Autodesk Fusion 360 part; units mm, degrees
(part 5 of 5)
sketch "Boceto9" plane through (0, 4.8, 0) normal (0, 1, 0) x (-1, 0, 0)
  line L0 (-13.4347, -89.9523) -> (-1.4347, -77.5976)
  arc A0 (1.4347, -77.5976) -> (-1.4347, -77.5976) centre (0, -78.991) ccw
  line L1 (1.4347, -77.5976) -> (13.4347, -89.9523)
  arc A1 (12, -93.3458) -> (13.4347, -89.9523) centre (12, -91.3458) ccw
  line L2 (12, -93.3458) -> (-12, -93.3458)
  arc A2 (-13.4347, -89.9523) -> (-12, -93.3458) centre (-12, -91.3458) ccw
  line L3 (13.0951, -76.1205) -> (19, -76.1205)
  arc A3 (21, -78.1205) -> (19, -76.1205) centre (19, -78.1205) ccw
  line L4 (21, -78.1205) -> (21, -84.2)
  arc A4 (17.5653, -85.5935) -> (21, -84.2) centre (19, -84.2) ccw
  line L5 (17.5653, -85.5935) -> (11.6604, -79.514)
  arc A5 (13.0951, -76.1205) -> (11.6604, -79.514) centre (13.0951, -78.1205) ccw
  line L6 (-11.6604, -79.514) -> (-17.5653, -85.5935)
  arc A6 (-21, -84.2) -> (-17.5653, -85.5935) centre (-19, -84.2) ccw
  line L7 (-21, -84.2) -> (-21, -78.1205)
  arc A7 (-19, -76.1205) -> (-21, -78.1205) centre (-19, -78.1205) ccw
  line L8 (-19, -76.1205) -> (-13.0951, -76.1205)
  arc A8 (-11.6604, -79.514) -> (-13.0951, -76.1205) centre (-13.0951, -78.1205) ccw
  line L9 (8, -66.3205) -> (8, -67.1205)
  arc A9 (5, -70.1205) -> (8, -67.1205) centre (5, -67.1205) ccw
  line L10 (5, -70.1205) -> (-5, -70.1205)
  arc A10 (-8, -67.1205) -> (-5, -70.1205) centre (-5, -67.1205) ccw
  line L11 (-8, -67.1205) -> (-8, -66.3205)
  arc A11 (-5, -63.3205) -> (-8, -66.3205) centre (-5, -66.3205) ccw
  line L12 (-5, -63.3205) -> (5, -63.3205)
  arc A12 (8, -66.3205) -> (5, -63.3205) centre (5, -66.3205) ccw
  circle A13 centre (138.0313, 4.5) radius 2.5
  circle A14 centre (-140.0313, 14.5) radius 4
  arc A15 (124.6679, -20.512) -> (128.2, -19.2264) centre (126.2, -19.2264) ccw
  line L13 (124.6679, -20.512) -> (114.4087, -8.2856)
  arc A16 (115.9408, -5) -> (114.4087, -8.2856) centre (115.9408, -7) ccw
  line L14 (115.9408, -5) -> (126.2, -5)
  arc A17 (128.2, -7) -> (126.2, -5) centre (126.2, -7) ccw
  line L15 (128.2, -7) -> (128.2, -19.2264)
  arc A18 (-114.4087, -8.2856) -> (-115.9408, -5) centre (-115.9408, -7) ccw
  line L16 (-114.4087, -8.2856) -> (-124.6679, -20.512)
  arc A19 (-128.2, -19.2264) -> (-124.6679, -20.512) centre (-126.2, -19.2264) ccw
  line L17 (-128.2, -19.2264) -> (-128.2, -7)
  arc A20 (-126.2, -5) -> (-128.2, -7) centre (-126.2, -7) ccw
  line L18 (-126.2, -5) -> (-115.9408, -5)
  circle A21 centre (-143.9289, -24) radius 2.5
  arc A22 (131.7, 16.1564) -> (129.934, 16.7992) centre (130.7, 16.1564) ccw
  line L19 (131.7, 16.1564) -> (131.7, 1)
  arc A23 (130.7, 0) -> (131.7, 1) centre (130.7, 1) ccw
  line L20 (130.7, 0) -> (117.9823, 0)
  arc A24 (117.2162, 1.6428) -> (117.9823, 0) centre (117.9823, 1) ccw
  line L21 (117.2162, 1.6428) -> (129.934, 16.7992)
  arc A25 (-129.934, 16.7992) -> (-131.7, 16.1564) centre (-130.7, 16.1564) ccw
  line L22 (-129.934, 16.7992) -> (-117.2162, 1.6428)
  arc A26 (-117.9823, 0) -> (-117.2162, 1.6428) centre (-117.9823, 1) ccw
  line L23 (-117.9823, 0) -> (-130.7, 0)
  arc A27 (-131.7, 1) -> (-130.7, 0) centre (-130.7, 1) ccw
  line L24 (-131.7, 1) -> (-131.7, 16.1564)
  circle A28 centre (143.9289, -24) radius 2.5
  circle A29 centre (-138.0313, 4.5) radius 2.5
  circle A30 centre (140.0313, 14.5) radius 4
  line L25 (23, -57.3205) -> (-23, -57.3205)
  line L26 (-23, -57.3205) -> (-23, -5)
  line L27 (-23, -5) -> (23, -5)
  line L28 (23, -5) -> (23, -57.3205)
  line L29 (30, -92.2) -> (122.2222, -25.3759)
  line L30 (122.2222, -25.3759) -> (126.7013, -30.7139)
  arc A31 (126.7013, -30.7139) -> (130.5315, -32.5) centre (130.5315, -27.5) ccw
  line L31 (130.5315, -32.5) -> (131.95, -32.5)
  line L32 (131.95, -32.5) -> (133.2, -31.25)
  line L33 (133.2, -31.25) -> (133.2, -5)
  line L34 (133.2, -5) -> (138, -5)
  line L35 (138, -5) -> (138, -31.5)
  line L36 (138, -31.5) -> (139, -32.5)
  line L37 (139, -32.5) -> (141.0289, -32.5)
  arc A32 (141.0289, -32.5) -> (149.6891, -17.5) centre (141.0289, -22.5) ccw
  arc A33 (148.5274, 15.3125) -> (149.6891, -17.5) centre (180, 0) ccw
  arc A34 (148.5274, 15.3125) -> (144.0313, 22.5) centre (144.0313, 17.5) ccw
  line L38 (144.0313, 22.5) -> (131.9209, 22.5)
  arc A35 (131.9209, 22.5) -> (125.7926, 19.6423) centre (131.9209, 14.5) ccw
  line L39 (125.7926, 19.6423) -> (115.9041, 7.8577)
  arc A36 (109.7758, 5) -> (115.9041, 7.8577) centre (109.7758, 13) ccw
  line L40 (109.7758, 5) -> (35, 5)
  arc A37 (30, 10) -> (35, 5) centre (35, 10) ccw
  line L41 (30, 10) -> (30, 12.6048)
  arc A38 (30, 12.6048) -> (26.8657, 15.6018) centre (27, 12.6048) ccw
  arc A39 (22.4813, 15.4213) -> (26.8657, 15.6018) centre (0, 615) ccw
  arc A40 (22.4813, 15.4213) -> (22, 14.9217) centre (22.5, 14.9217) ccw
  line L42 (22, 14.9217) -> (22, 8)
  line L43 (22, 8) -> (17.2, 8)
  line L44 (17.2, 8) -> (17.2, 14.7323)
  arc A41 (17.2, 14.7323) -> (16.6861, 15.2321) centre (16.7, 14.7323) ccw
  arc A42 (-8.6105, 15.0618) -> (16.6861, 15.2321) centre (0, 615) ccw
  line L45 (-8.6105, 15.0618) -> (-4.2286, 3.0227)
  arc A43 (-4.2286, 3.0227) -> (0, 9.0618) centre (0, 4.5618) ccw
  arc A44 (0, 11.0618) -> (0, 9.0618) centre (0, 10.0618) ccw
  arc A45 (-6.108, 2.3387) -> (0, 11.0618) centre (0, 4.5618) ccw
  line L46 (-6.108, 2.3387) -> (-10.7514, 15.0963)
  arc A46 (-16.6861, 15.2321) -> (-10.7514, 15.0963) centre (0, 615) ccw
  arc A47 (-16.6861, 15.2321) -> (-17.2, 14.7323) centre (-16.7, 14.7323) ccw
  line L47 (-17.2, 14.7323) -> (-17.2, 8)
  line L48 (-17.2, 8) -> (-22, 8)
  line L49 (-22, 8) -> (-22, 14.9217)
  arc A48 (-22, 14.9217) -> (-22.4813, 15.4213) centre (-22.5, 14.9217) ccw
  arc A49 (-26.8657, 15.6018) -> (-22.4813, 15.4213) centre (0, 615) ccw
  arc A50 (-26.8657, 15.6018) -> (-30, 12.6048) centre (-27, 12.6048) ccw
  line L50 (-30, 12.6048) -> (-30, 10)
  arc A51 (-35, 5) -> (-30, 10) centre (-35, 10) ccw
  line L51 (-35, 5) -> (-109.7758, 5)
  arc A52 (-115.9041, 7.8577) -> (-109.7758, 5) centre (-109.7758, 13) ccw
  line L52 (-115.9041, 7.8577) -> (-125.7926, 19.6423)
  arc A53 (-125.7926, 19.6423) -> (-131.9209, 22.5) centre (-131.9209, 14.5) ccw
  line L53 (-131.9209, 22.5) -> (-144.0313, 22.5)
  arc A54 (-144.0313, 22.5) -> (-148.5274, 15.3125) centre (-144.0313, 17.5) ccw
  arc A55 (-149.6891, -17.5) -> (-148.5274, 15.3125) centre (-180, 0) ccw
  arc A56 (-149.6891, -17.5) -> (-141.0289, -32.5) centre (-141.0289, -22.5) ccw
  line L54 (-141.0289, -32.5) -> (-139, -32.5)
  line L55 (-139, -32.5) -> (-138, -31.5)
  line L56 (-138, -31.5) -> (-138, -5)
  line L57 (-138, -5) -> (-133.2, -5)
  line L58 (-133.2, -5) -> (-133.2, -31.25)
  line L59 (-133.2, -31.25) -> (-131.95, -32.5)
  line L60 (-131.95, -32.5) -> (-130.5315, -32.5)
  arc A57 (-130.5315, -32.5) -> (-126.7013, -30.7139) centre (-130.5315, -27.5) ccw
  line L61 (-126.7013, -30.7139) -> (-122.2222, -25.3759)
  line L62 (-122.2222, -25.3759) -> (-30, -92.2)
  line L63 (-30, -92.2) -> (-20, -92.2)
  line L64 (-20, -92.2) -> (-20, -97)
  line L65 (-20, -97) -> (-30, -97)
  line L66 (-30, -97) -> (-30, -101)
  arc A58 (-30, -101) -> (-26, -105) centre (-26, -101) ccw
  line L67 (-26, -105) -> (-10, -105)
  line L68 (-10, -105) -> (-0.8439, -100.7385)
  arc A59 (0.8439, -100.7385) -> (-0.8439, -100.7385) centre (0, -102.5518) ccw
  line L69 (0.8439, -100.7385) -> (10, -105)
  line L70 (10, -105) -> (26, -105)
  arc A60 (26, -105) -> (30, -101) centre (26, -101) ccw
  line L71 (30, -101) -> (30, -97)
  line L72 (30, -97) -> (20, -97)
  line L73 (20, -97) -> (20, -92.2)
  line L74 (20, -92.2) -> (30, -92.2)
  line L75 (30, -63.3205) -> (30, -7.5)
  arc A61 (32.5, -5) -> (30, -7.5) centre (32.5, -7.5) ccw
  line L76 (32.5, -5) -> (101.3943, -5)
  arc A62 (107.5227, -7.8577) -> (101.3943, -5) centre (101.3943, -13) ccw
  line L77 (107.5227, -7.8577) -> (117.7113, -20)
  line L78 (117.7113, -20) -> (30, -83.5555)
  line L79 (30, -83.5555) -> (30, -68.1205)
  line L80 (30, -68.1205) -> (16, -68.1205)
  line L81 (16, -68.1205) -> (16, -63.3205)
  line L82 (16, -63.3205) -> (30, -63.3205)
  line L83 (-30, -7.5) -> (-30, -63.3205)
  line L84 (-30, -63.3205) -> (-16, -63.3205)
  line L85 (-16, -63.3205) -> (-16, -68.1205)
  line L86 (-16, -68.1205) -> (-30, -68.1205)
  line L87 (-30, -68.1205) -> (-30, -83.5555)
  line L88 (-30, -83.5555) -> (-117.7113, -20)
  line L89 (-117.7113, -20) -> (-107.5227, -7.8577)
  arc A63 (-101.3943, -5) -> (-107.5227, -7.8577) centre (-101.3943, -13) ccw
  line L90 (-101.3943, -5) -> (-32.5, -5)
  arc A64 (-30, -7.5) -> (-32.5, -5) centre (-32.5, -7.5) ccw
  line L91 (-30, -63.3205) -> (-88.3205, -5)
  line L92 (-30, -52.0068) -> (-77.0068, -5)
  line L93 (0, 1.75) -> (0, 22.5)
  line L94 (30, -52.0068) -> (77.0068, -5)
  line L95 (30, -63.3205) -> (88.3205, -5)
  dimension "d158" = 8
  dimension "d159" = 45
  constraint coincident L83.end L84.start
  constraint coincident L90 L91.end
  constraint coincident L83 L92.start
  constraint coincident L90 L92.end
  constraint parallel L91 L92
  constraint symmetric L83.end L93 L75.start
  constraint symmetric L91.end L93 L95.end
  constraint symmetric L92.start L93 L94.start
  constraint symmetric L92.end L93 L94.end
  measures "d158" distance of L91 L92
  measures "d159" angle of L83 L92
extrude "Extruir8" add sketch "Boceto9" against normal blind 4.8 contours L75 L76 L94 L95 | L83 L90 L91 L92
chamfer "Chaflán3" distance 5 angle 45 4 edges at (23, 2.4, -57.3205) (23, 2.4, -5) (-23, 2.4, -57.3205) (-23, 2.4, -5)
fillet "Empalme7" radius 5 12 edges at (30, 2.4, -83.5555) (30, 2.4, -52.0068) (77.0068, 2.4, -5) (122.2222, 2.4, -25.3759) (117.7113, 2.4, -20) (-30, 2.4, -83.5555) (-30, 2.4, -52.0068) (-77.0068, 2.4, -5) (-117.7113, 2.4, -20) (-122.2222, 2.4, -25.3759) (-88.3205, 2.4, -5) (88.3205, 2.4, -5)
chamfer "Chaflán4" distance 1 angle 45 7 edges at (30, 2.4, -68.1205) (30, 2.4, -97) (-30, 2.4, -97) (-30, 2.4, -68.1205) (8.6105, 2.4, 15.0618) (30, 2.4, -63.3205) (-30, 2.4, -63.3205)
sketch "Boceto11" plane through (0, 4.8, 0) normal (0, 1, 0) x (-1, 0, 0)
  line L0 (29, -63.3205) -> (30.7071, -62.6134)
  line L1 (30.7071, -62.6134) -> (86.856, -6.4645)
  arc A0 (90.3916, -5) -> (86.856, -6.4645) centre (90.3916, -10) ccw
  line L2 (90.3916, -5) -> (101.3943, -5)
  arc A1 (107.5227, -7.8577) -> (101.3943, -5) centre (101.3943, -13) ccw
  line L3 (107.5227, -7.8577) -> (114.2603, -15.8873)
  arc A2 (113.3639, -23.1501) -> (114.2603, -15.8873) centre (110.4301, -19.1013) ccw
  line L4 (113.3639, -23.1501) -> (37.9338, -77.8067)
  arc A3 (30, -73.7579) -> (37.9338, -77.8067) centre (35, -73.7579) ccw
  line L5 (30, -73.7579) -> (30, -69.1205)
  line L6 (30, -69.1205) -> (29, -68.1205)
  line L7 (29, -68.1205) -> (16, -68.1205)
  line L8 (16, -68.1205) -> (16, -63.3205)
  line L9 (16, -63.3205) -> (29, -63.3205)
  line L10 (-30.7071, -62.6134) -> (-29, -63.3205)
  line L11 (-29, -63.3205) -> (-16, -63.3205)
  line L12 (-16, -63.3205) -> (-16, -68.1205)
  line L13 (-16, -68.1205) -> (-29, -68.1205)
  line L14 (-29, -68.1205) -> (-30, -69.1205)
  line L15 (-30, -69.1205) -> (-30, -73.7579)
  arc A4 (-37.9338, -77.8067) -> (-30, -73.7579) centre (-35, -73.7579) ccw
  line L16 (-37.9338, -77.8067) -> (-113.3639, -23.1501)
  arc A5 (-114.2603, -15.8873) -> (-113.3639, -23.1501) centre (-110.4301, -19.1013) ccw
  line L17 (-114.2603, -15.8873) -> (-107.5227, -7.8577)
  arc A6 (-101.3943, -5) -> (-107.5227, -7.8577) centre (-101.3943, -13) ccw
  line L18 (-101.3943, -5) -> (-90.3916, -5)
  arc A7 (-86.856, -6.4645) -> (-90.3916, -5) centre (-90.3916, -10) ccw
  line L19 (-86.856, -6.4645) -> (-30.7071, -62.6134)
  line L20 (30, -39.9357) -> (30, -7.5)
  arc A8 (32.5, -5) -> (30, -7.5) centre (32.5, -7.5) ccw
  line L21 (32.5, -5) -> (64.9357, -5)
  arc A9 (68.4713, -13.5355) -> (64.9357, -5) centre (64.9357, -10) ccw
  line L22 (68.4713, -13.5355) -> (38.5355, -43.4713)
  arc A10 (30, -39.9357) -> (38.5355, -43.4713) centre (35, -39.9357) ccw
  line L23 (18, -57.3205) -> (-18, -57.3205)
  line L24 (-18, -57.3205) -> (-23, -52.3205)
  line L25 (-23, -52.3205) -> (-23, -10)
  line L26 (-23, -10) -> (-18, -5)
  line L27 (-18, -5) -> (18, -5)
  line L28 (18, -5) -> (23, -10)
  line L29 (23, -10) -> (23, -52.3205)
  line L30 (23, -52.3205) -> (18, -57.3205)
  circle A11 centre (140.0313, 14.5) radius 4
  arc A12 (124.6679, -20.512) -> (128.2, -19.2264) centre (126.2, -19.2264) ccw
  line L31 (124.6679, -20.512) -> (114.4087, -8.2856)
  arc A13 (115.9408, -5) -> (114.4087, -8.2856) centre (115.9408, -7) ccw
  line L32 (115.9408, -5) -> (126.2, -5)
  arc A14 (128.2, -7) -> (126.2, -5) centre (126.2, -7) ccw
  line L33 (128.2, -7) -> (128.2, -19.2264)
  arc A15 (131.7, 16.1564) -> (129.934, 16.7992) centre (130.7, 16.1564) ccw
  line L34 (131.7, 16.1564) -> (131.7, 1)
  arc A16 (130.7, 0) -> (131.7, 1) centre (130.7, 1) ccw
  line L35 (130.7, 0) -> (117.9823, 0)
  arc A17 (117.2162, 1.6428) -> (117.9823, 0) centre (117.9823, 1) ccw
  line L36 (117.2162, 1.6428) -> (129.934, 16.7992)
  circle A18 centre (-143.9289, -24) radius 2.5
  circle A19 centre (-140.0313, 14.5) radius 4
  circle A20 centre (143.9289, -24) radius 2.5
  circle A21 centre (-138.0313, 4.5) radius 2.5
  arc A22 (-129.934, 16.7992) -> (-131.7, 16.1564) centre (-130.7, 16.1564) ccw
  line L37 (-129.934, 16.7992) -> (-117.2162, 1.6428)
  arc A23 (-117.9823, 0) -> (-117.2162, 1.6428) centre (-117.9823, 1) ccw
  line L38 (-117.9823, 0) -> (-130.7, 0)
  arc A24 (-131.7, 1) -> (-130.7, 0) centre (-130.7, 1) ccw
  line L39 (-131.7, 1) -> (-131.7, 16.1564)
  circle A25 centre (138.0313, 4.5) radius 2.5
  arc A26 (-114.4087, -8.2856) -> (-115.9408, -5) centre (-115.9408, -7) ccw
  line L40 (-114.4087, -8.2856) -> (-124.6679, -20.512)
  arc A27 (-128.2, -19.2264) -> (-124.6679, -20.512) centre (-126.2, -19.2264) ccw
  line L41 (-128.2, -19.2264) -> (-128.2, -7)
  arc A28 (-126.2, -5) -> (-128.2, -7) centre (-126.2, -7) ccw
  line L42 (-126.2, -5) -> (-115.9408, -5)
  line L43 (8, -66.3205) -> (8, -67.1205)
  arc A29 (5, -70.1205) -> (8, -67.1205) centre (5, -67.1205) ccw
  line L44 (5, -70.1205) -> (-5, -70.1205)
  arc A30 (-8, -67.1205) -> (-5, -70.1205) centre (-5, -67.1205) ccw
  line L45 (-8, -67.1205) -> (-8, -66.3205)
  arc A31 (-5, -63.3205) -> (-8, -66.3205) centre (-5, -66.3205) ccw
  line L46 (-5, -63.3205) -> (5, -63.3205)
  arc A32 (8, -66.3205) -> (5, -63.3205) centre (5, -66.3205) ccw
  line L47 (-11.6604, -79.514) -> (-17.5653, -85.5935)
  arc A33 (-21, -84.2) -> (-17.5653, -85.5935) centre (-19, -84.2) ccw
  line L48 (-21, -84.2) -> (-21, -78.1205)
  arc A34 (-19, -76.1205) -> (-21, -78.1205) centre (-19, -78.1205) ccw
  line L49 (-19, -76.1205) -> (-13.0951, -76.1205)
  arc A35 (-11.6604, -79.514) -> (-13.0951, -76.1205) centre (-13.0951, -78.1205) ccw
  line L50 (13.0951, -76.1205) -> (19, -76.1205)
  arc A36 (21, -78.1205) -> (19, -76.1205) centre (19, -78.1205) ccw
  line L51 (21, -78.1205) -> (21, -84.2)
  arc A37 (17.5653, -85.5935) -> (21, -84.2) centre (19, -84.2) ccw
  line L52 (17.5653, -85.5935) -> (11.6604, -79.514)
  arc A38 (13.0951, -76.1205) -> (11.6604, -79.514) centre (13.0951, -78.1205) ccw
  line L53 (-13.4347, -89.9523) -> (-1.4347, -77.5976)
  arc A39 (1.4347, -77.5976) -> (-1.4347, -77.5976) centre (0, -78.991) ccw
  line L54 (1.4347, -77.5976) -> (13.4347, -89.9523)
  arc A40 (12, -93.3458) -> (13.4347, -89.9523) centre (12, -91.3458) ccw
  line L55 (12, -93.3458) -> (-12, -93.3458)
  arc A41 (-13.4347, -89.9523) -> (-12, -93.3458) centre (-12, -91.3458) ccw
  line L56 (-64.9357, -5) -> (-32.5, -5)
  arc A42 (-30, -7.5) -> (-32.5, -5) centre (-32.5, -7.5) ccw
  line L57 (-30, -7.5) -> (-30, -39.9357)
  arc A43 (-38.5355, -43.4713) -> (-30, -39.9357) centre (-35, -39.9357) ccw
  line L58 (-38.5355, -43.4713) -> (-68.4713, -13.5355)
  arc A44 (-64.9357, -5) -> (-68.4713, -13.5355) centre (-64.9357, -10) ccw
  line L59 (-7.6106, 15.0483) -> (-8.2685, 14.1221)
  line L60 (-8.2685, 14.1221) -> (-4.2286, 3.0227)
  arc A45 (-4.2286, 3.0227) -> (0, 9.0618) centre (0, 4.5618) ccw
  arc A46 (0, 11.0618) -> (0, 9.0618) centre (0, 10.0618) ccw
  arc A47 (-6.108, 2.3387) -> (0, 11.0618) centre (0, 4.5618) ccw
  line L61 (-6.108, 2.3387) -> (-10.7514, 15.0963)
  arc A48 (-16.6861, 15.2321) -> (-10.7514, 15.0963) centre (0, 615) ccw
  arc A49 (-16.6861, 15.2321) -> (-17.2, 14.7323) centre (-16.7, 14.7323) ccw
  line L62 (-17.2, 14.7323) -> (-17.2, 8)
  line L63 (-17.2, 8) -> (-22, 8)
  line L64 (-22, 8) -> (-22, 14.9217)
  arc A50 (-22, 14.9217) -> (-22.4813, 15.4213) centre (-22.5, 14.9217) ccw
  arc A51 (-26.8657, 15.6018) -> (-22.4813, 15.4213) centre (0, 615) ccw
  arc A52 (-26.8657, 15.6018) -> (-30, 12.6048) centre (-27, 12.6048) ccw
  line L65 (-30, 12.6048) -> (-30, 10)
  arc A53 (-35, 5) -> (-30, 10) centre (-35, 10) ccw
  line L66 (-35, 5) -> (-109.7758, 5)
  arc A54 (-115.9041, 7.8577) -> (-109.7758, 5) centre (-109.7758, 13) ccw
  line L67 (-115.9041, 7.8577) -> (-125.7926, 19.6423)
  arc A55 (-125.7926, 19.6423) -> (-131.9209, 22.5) centre (-131.9209, 14.5) ccw
  line L68 (-131.9209, 22.5) -> (-144.0313, 22.5)
  arc A56 (-144.0313, 22.5) -> (-148.5274, 15.3125) centre (-144.0313, 17.5) ccw
  arc A57 (-149.6891, -17.5) -> (-148.5274, 15.3125) centre (-180, 0) ccw
  arc A58 (-149.6891, -17.5) -> (-141.0289, -32.5) centre (-141.0289, -22.5) ccw
  line L69 (-141.0289, -32.5) -> (-139, -32.5)
  line L70 (-139, -32.5) -> (-138, -31.5)
  line L71 (-138, -31.5) -> (-138, -5)
  line L72 (-138, -5) -> (-133.2, -5)
  line L73 (-133.2, -5) -> (-133.2, -31.25)
  line L74 (-133.2, -31.25) -> (-131.95, -32.5)
  line L75 (-131.95, -32.5) -> (-130.5315, -32.5)
  arc A59 (-130.5315, -32.5) -> (-126.7013, -30.7139) centre (-130.5315, -27.5) ccw
  line L76 (-126.7013, -30.7139) -> (-125.2154, -28.9431)
  arc A60 (-118.4514, -28.1082) -> (-125.2154, -28.9431) centre (-121.3852, -32.157) ccw
  line L77 (-118.4514, -28.1082) -> (-30, -92.2)
  line L78 (-30, -92.2) -> (-20, -92.2)
  line L79 (-20, -92.2) -> (-20, -97)
  line L80 (-20, -97) -> (-29, -97)
  line L81 (-29, -97) -> (-30, -98)
  line L82 (-30, -98) -> (-30, -101)
  arc A61 (-30, -101) -> (-26, -105) centre (-26, -101) ccw
  line L83 (-26, -105) -> (-10, -105)
  line L84 (-10, -105) -> (-0.8439, -100.7385)
  arc A62 (0.8439, -100.7385) -> (-0.8439, -100.7385) centre (0, -102.5518) ccw
  line L85 (0.8439, -100.7385) -> (10, -105)
  line L86 (10, -105) -> (26, -105)
  arc A63 (26, -105) -> (30, -101) centre (26, -101) ccw
  line L87 (30, -101) -> (30, -98)
  line L88 (30, -98) -> (29, -97)
  line L89 (29, -97) -> (20, -97)
  line L90 (20, -97) -> (20, -92.2)
  line L91 (20, -92.2) -> (30, -92.2)
  line L92 (30, -92.2) -> (118.4514, -28.1082)
  arc A64 (125.2154, -28.9431) -> (118.4514, -28.1082) centre (121.3852, -32.157) ccw
  line L93 (125.2154, -28.9431) -> (126.7013, -30.7139)
  arc A65 (126.7013, -30.7139) -> (130.5315, -32.5) centre (130.5315, -27.5) ccw
  line L94 (130.5315, -32.5) -> (131.95, -32.5)
  line L95 (131.95, -32.5) -> (133.2, -31.25)
  line L96 (133.2, -31.25) -> (133.2, -5)
  line L97 (133.2, -5) -> (138, -5)
  line L98 (138, -5) -> (138, -31.5)
  line L99 (138, -31.5) -> (139, -32.5)
  line L100 (139, -32.5) -> (141.0289, -32.5)
  arc A66 (141.0289, -32.5) -> (149.6891, -17.5) centre (141.0289, -22.5) ccw
  arc A67 (148.5274, 15.3125) -> (149.6891, -17.5) centre (180, 0) ccw
  arc A68 (148.5274, 15.3125) -> (144.0313, 22.5) centre (144.0313, 17.5) ccw
  line L101 (144.0313, 22.5) -> (131.9209, 22.5)
  arc A69 (131.9209, 22.5) -> (125.7926, 19.6423) centre (131.9209, 14.5) ccw
  line L102 (125.7926, 19.6423) -> (115.9041, 7.8577)
  arc A70 (109.7758, 5) -> (115.9041, 7.8577) centre (109.7758, 13) ccw
  line L103 (109.7758, 5) -> (35, 5)
  arc A71 (30, 10) -> (35, 5) centre (35, 10) ccw
  line L104 (30, 10) -> (30, 12.6048)
  arc A72 (30, 12.6048) -> (26.8657, 15.6018) centre (27, 12.6048) ccw
  arc A73 (22.4813, 15.4213) -> (26.8657, 15.6018) centre (0, 615) ccw
  arc A74 (22.4813, 15.4213) -> (22, 14.9217) centre (22.5, 14.9217) ccw
  line L105 (22, 14.9217) -> (22, 8)
  line L106 (22, 8) -> (17.2, 8)
  line L107 (17.2, 8) -> (17.2, 14.7323)
  arc A75 (17.2, 14.7323) -> (16.6861, 15.2321) centre (16.7, 14.7323) ccw
  arc A76 (-7.6106, 15.0483) -> (16.6861, 15.2321) centre (0, 615) ccw
equation "d8 = d7 / 2"
equation "d28 = d23"
equation "d32 = 27.5 mm + 5 mm"
equation "d45 = d44"
equation "d47 = d46"
equation "d51 = 60 mm"
equation "d52 = d51 / 2"
equation "d65 = d67"
equation "d102 = d103"
equation "d112 = d102"
equation "d152 = d153"

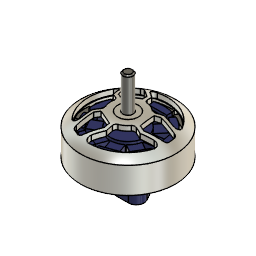
design "1102 BRUSHLESS"
Autodesk Fusion 360 part; units mm, degrees
sketch "Boceto1" plane through (0, 0, 0) normal (0, 0, 1) x (1, 0, 0)
  line L0 (-3.847, -1.0789) -> (-0.9891, 3.8711)
  line L1 (0.9891, 3.8711) -> (3.847, -1.0789)
  line L2 (2.8579, -2.7921) -> (-2.8579, -2.7921)
  line L3 (0, -2.7921) -> (0, 5.9712) construction
  line L4 (-2.5255, 1.2099) -> (5.4503, -2.6111) construction
  circle A0 centre (0, 3.3) radius 0.7
  circle A1 centre (0, 0) radius 3.3 construction
  arc A2 (0.9891, 3.8711) -> (-0.9891, 3.8711) centre (0, 3.3) ccw
  circle A3 centre (-2.8579, -1.65) radius 0.7
  arc A4 (-3.847, -1.0789) -> (-2.8579, -2.7921) centre (-2.8579, -1.65) ccw
  circle A5 centre (2.8579, -1.65) radius 0.7
  arc A6 (2.8579, -2.7921) -> (3.847, -1.0789) centre (2.8579, -1.65) ccw
  line L5 (-4, -1.65) -> (4, -1.65) construction
  line L6 (4, -1.65) -> (4, -0.8) construction
  dimension "d3" = 6.6
  dimension "d4" = 1.4
  dimension "d7" = 360
  dimension "d8" = 8
  constraint horizontal L2
  constraint vertical L3
  constraint coincident A1.centre L3
  constraint coincident A1.centre L4
  constraint coincident L3 A0.centre
  constraint coincident A1.centre origin
  constraint coincident A0.centre A1
  constraint tangent L1 A2
  constraint coincident L0 L4.start
  constraint concentric A0 A2
  constraint coincident A4 L2.end
  constraint coincident L2 L3.start
  constraint coincident A6 L2.start
  constraint coincident L1.end A6.end
  constraint tangent L0 A2
  constraint coincident A4 L5.start
  constraint coincident A6 L5.end
  constraint horizontal L5
  constraint coincident L2.start A6.start
  constraint perpendicular L5 L6
  constraint tangent A6 L6
  measures "d3" diameter of A1
  measures "d4" diameter of A0
  measures "d8" distance of L5.start L5.end
extrude "Extruir1" add sketch "Boceto1" along normal blind 1.25 makes body 1
sketch "Boceto2" plane through (0, 0, 1.25) normal (0, 0, 1) x (-1, 0, 0)
  circle A0 centre (2.8579, 1.65) radius 0.7
  circle A1 centre (0, -3.3) radius 0.7
  circle A2 centre (-2.8579, 1.65) radius 0.7
  arc A3 (3.847, 1.0789) -> (2.8579, 2.7921) centre (2.8579, 1.65) ccw
  line L0 (2.8579, 2.7921) -> (-2.8579, 2.7921)
  arc A4 (-2.8579, 2.7921) -> (-3.847, 1.0789) centre (-2.8579, 1.65) ccw
  line L1 (-3.847, 1.0789) -> (-0.9891, -3.8711)
  arc A5 (-0.9891, -3.8711) -> (0.9891, -3.8711) centre (0, -3.3) ccw
  line L2 (0.9891, -3.8711) -> (3.847, 1.0789)
  circle A6 centre (0, 0) radius 2.6
  constraint coincident A6.centre origin
  constraint tangent A1 A6
extrude "Extruir2" add sketch "Boceto2" along normal blind 5.5 contours A6 bodies 1
sketch "Boceto3" plane through (0, 0, 0) normal (0, 0, -1) x (1, 0, 0)
  circle A0 centre (-2.8579, 1.65) radius 0.7
  circle A1 centre (0, -3.3) radius 0.7
  circle A2 centre (2.8579, 1.65) radius 0.7
  arc A3 (-2.8579, 2.7921) -> (-3.847, 1.0789) centre (-2.8579, 1.65) ccw
  line L0 (-3.847, 1.0789) -> (-0.9891, -3.8711)
  arc A4 (-0.9891, -3.8711) -> (0.9891, -3.8711) centre (0, -3.3) ccw
  line L1 (0.9891, -3.8711) -> (3.847, 1.0789)
  arc A5 (3.847, 1.0789) -> (2.8579, 2.7921) centre (2.8579, 1.65) ccw
  line L2 (2.8579, 2.7921) -> (-2.8579, 2.7921)
  circle A6 centre (0, 0) radius 2
  dimension "d14" = 4
  constraint coincident A6.centre origin
  measures "d14" diameter of A6
extrude "Extruir3" cut sketch "Boceto3" against normal blind 1 contours A6 bodies 1
sketch "Boceto4" plane through (0, 0, 1) normal (0, 0, -1) x (1, 0, 0)
  circle A0 centre (0, 0) radius 2
  circle A1 centre (0, 0) radius 0.75
  dimension "d17" = 1.5
  constraint coincident A0.centre A1.centre
  measures "d17" diameter of A1
extrude "Extruir4" cut sketch "Boceto4" against normal blind 10 contours A1 bodies 1
extrude "Extruir5" add 1 faces at (1.5731, 0.1366, 1) along direction (0, 0, -1) blind 1 separate body on bodies 1 makes body 2
sketch "Boceto5" plane through (0, 0, 0) normal (0, 0, -1) x (1, 0, 0)
  circle A0 centre (0, 0) radius 0.75
  circle A1 centre (0, 0) radius 2
extrude "Extruir6" add sketch "Boceto5" against normal blind 13.75 separate body contours A0 makes body 3
extrude "Extruir8" add 1 faces at (0.5555, 0.0837, 0) along direction (0, 0, -1) blind 0.5 on bodies 3 bodies 3
ref_plane "PlanoDeObra1" through (0, 2.6, 5.2604) normal (0, 1, 0) x (1, 0, 0)
sketch "Boceto7" plane through (0, 2.6, 0) normal (0, 1, 0) x (1, 0, 0)
  line L0 (0.85, -6.35) -> (-0.85, -6.35)
  line L1 (-0.85, -6.35) -> (-0.85, -4.05)
  line L2 (-0.85, -4.05) -> (0.85, -4.05)
  line L3 (0.85, -4.05) -> (0.85, -6.35)
  line L4 (-2.6, -6.75) -> (2.6, -6.75)
  line L5 (0, -4.05) -> (0, -6.35) construction
  dimension "d30" = 1.7
  dimension "d31" = 2.3
  dimension "d42" = 0.4
  constraint horizontal L0
  constraint vertical L1
  constraint horizontal L2
  constraint vertical L3
  constraint midpoint L2 L5.start
  constraint midpoint L0 L5.end
  constraint coincident origin L5
  constraint coincident L0.end L1.start
  measures "d30" distance of L0.start L0.end
  measures "d31" distance of L0.start L2.end
  measures "d42" distance of L0 L4
extrude "Extruir9" add sketch "Boceto7" along normal blind 1.7 and the other way blind 0.5 bodies 1
sketch "Boceto8" plane through (0, 4.3, 0) normal (0, 1, 0) x (-1, 0, 0)
  line L0 (0.85, 6.35) -> (-0.85, 6.35)
  line L1 (-0.85, 6.35) -> (-0.85, 4.05)
  line L2 (-0.85, 4.05) -> (0.85, 4.05)
  line L3 (0.85, 4.05) -> (0.85, 6.35)
  line L4 (1.35, 3.65) -> (1.35, 6.75)
  line L5 (-1.35, 6.75) -> (-1.35, 3.65)
  line L6 (-1.35, 6.75) -> (1.35, 6.75)
  line L7 (2.6, 6.75) -> (-2.6, 6.75)
  line L8 (-1.35, 3.65) -> (1.35, 3.65)
  dimension "d36" = 2.7
  dimension "d37" = 1.35
  dimension "d43" = 0.4
  constraint vertical L4
  constraint vertical L5
  constraint perpendicular L4 L6
  constraint coincident L4.end L7
  constraint perpendicular L4 L8
  measures "d36" distance of L5.end L4.start
  measures "d37" distance of origin L5
  measures "d43" distance of L2 L8
extrude "Extruir10" add sketch "Boceto8" along normal blind 1 contours L0 L1 L2 L3 | L4 L5 L6 L7 L8 bodies 1
pattern_circular "Patrón C1" count 9 over 360 about axis through (0, 0, 1) along (0, 0, 1) of "Extruir9", "Extruir10"
sketch "Boceto9" plane through (0, 0, 6.75) normal (0, 0, 1) x (-1, 0, 0)
  circle A0 centre (0, 0) radius 0.75
  circle A1 centre (0, 0) radius 2.6
  circle A2 centre (0, 0) radius 5.25
  circle A3 centre (0, 0) radius 7.25
  dimension "d44" = 10.5
  dimension "d45" = 2
  constraint coincident A0.centre A1.centre
  measures "d44" diameter of A2
extrude "Extruir11" cut sketch "Boceto9" against normal blind 3.1 contours A3 bodies 1
ref_plane "PlanoDeObra2" through (0, 0.825, 3) normal (0, 0, -1) x (-1, 0, 0)
sketch "Boceto10" plane through (0, 0, 3) normal (0, 0, -1) x (-1, 0, 0)
  circle A0 centre (0, 0) radius 6.9
  circle A1 centre (0, 0) radius 6.2
  dimension "d50" = 13.8
  dimension "d51" = -0.7
  constraint coincident A0.centre A1.centre
  measures "d50" diameter of A0
extrude "Extruir12" add sketch "Boceto10" against normal blind 3.8 separate body makes body 4
ref_plane "PlanoDeObra3" through (0, -6.2, 4.5387) normal (0, 1, 0) x (1, 0, 0)
sketch "Boceto11" plane through (0, -6.2, 0) normal (0, 1, 0) x (1, 0, 0)
  line L0 (1.25, -3) -> (-1.25, -3)
  line L1 (-1.25, -3) -> (-1.25, -6)
  line L2 (-1.25, -6) -> (1.25, -6)
  line L3 (1.25, -6) -> (1.25, -3)
  line L4 (-6.2, -3) -> (6.2, -3)
  dimension "d56" = 2.5
  dimension "d57" = 3
  dimension "d58" = 1.25
  constraint horizontal L0
  constraint vertical L1
  constraint horizontal L2
  constraint vertical L3
  constraint coincident L0.end L4
  measures "d56" distance of L1.end L2.end
  measures "d57" distance of L0.end L1.end
  measures "d58" distance of origin L1
extrude "Extruir13" add sketch "Boceto11" along normal blind 0.7 separate body makes body 5
pattern_circular "Patrón C2" count 12 over 360 about axis through (0, 0, -0.5) along (0, 0, 1) of "Extruir13" makes body 6 at (2.7392, -5.5777, 5) makes body 7 at (5.161, -3.4608, 4) makes body 8 at (6.2, 0.4167, 5) makes body 9 at (4.9715, 2.3892, 4) makes body 10 at (3.1108, 4.5548, 4) makes body 11 at (-0.4167, 6.2, 5) makes body 12 at (-2.7392, 5.5777, 4) makes body 13 at (-5.5777, 2.7392, 4) makes body 14 at (-6.2, -0.4167, 5) makes body 15 at (-5.5777, -2.7392, 4) makes body 16 at (-2.7392, -5.5777, 5)
sketch "Boceto14" plane through (0, 0, 0) normal (1, 0, 0) x (0, 1, 0)
  line L0 (0, 8.75) -> (1.5, 8.75)
  arc A0 (6.9, 6.8) -> (1.5, 8.75) centre (1.5, 0.2981) ccw
  line L1 (6.9, 6.8) -> (-6.9, 6.8)
  line L2 (0, 8.75) -> (0, 6.8)
  line L3 (0, 8.05) -> (1.5, 8.05)
  arc A1 (5.7211, 6.8) -> (1.5, 8.05) centre (1.5, 0.2981) ccw
  dimension "d68" = 3
  dimension "d69" = 1.95
  constraint horizontal L0
  constraint tangent L0 A0
  constraint coincident A0.start L1
  constraint midpoint L1 L2.end
  constraint perpendicular L1 L2
  constraint coincident A0.start L1.start
  constraint coincident L2 L3.start
  constraint concentric A0 A1
  constraint tangent L3 A1
  constraint coincident L1 A1.start
  measures "d69" distance of L0.start L2.end
revolve "Revolución1" add sketch "Boceto14" angle 360 about axis through (0, 0, 8.75) along (0, 0, -1) contours L0 A0 L1 L2 L3 A1 bodies 4
sketch "Boceto15" plane through (0, 0, 8.75) normal (0, 0, 1) x (-1, 0, 0)
  circle A0 centre (0, 0) radius 1.5
  circle A1 centre (0, 0) radius 0.75
  circle A2 centre (0, 0) radius 5.75
  circle A3 centre (0, 0) radius 6.9
  circle A4 centre (0, 0) radius 2.5
  line L0 (-1.3525, -5.5887) -> (-2, -3.1721)
  line L1 (0, 0) -> (0, -5.75) construction
  line L2 (-2, -3.1721) -> (-1.4653, -2.0255)
  circle A5 centre (0, 0) radius 3.75 construction
  line L3 (-1.4653, -2.0255) -> (0, -2.0255)
  line L4 (1.4653, -2.0255) -> (0, -2.0255)
  line L5 (2, -3.1721) -> (1.4653, -2.0255)
  line L6 (1.3525, -5.5887) -> (2, -3.1721)
  line L7 (0.8069, -5.6931) -> (1.4699, -3.2185)
  line L8 (1.4699, -3.2185) -> (1.1468, -2.5255)
  line L9 (1.1468, -2.5255) -> (0, -2.5255)
  line L10 (-1.1468, -2.5255) -> (0, -2.5255)
  line L11 (-1.4699, -3.2185) -> (-1.1468, -2.5255)
  line L12 (-0.8069, -5.6931) -> (-1.4699, -3.2185)
  line L13 (5.5162, 1.623) -> (3.7472, -0.146)
  line L14 (5.3338, 2.1478) -> (3.5223, 0.3363)
  line L15 (3.5223, 0.3363) -> (2.7606, 0.2696)
  line L16 (1.6138, 2.2559) -> (2.1872, 1.2628)
  line L17 (2.7606, 0.2696) -> (2.1872, 1.2628)
  line L18 (3.7472, -0.146) -> (2.4868, -0.2562)
  line L19 (4.5269, 3.5453) -> (2.0524, 2.8823)
  line L20 (4.1637, 3.9656) -> (1.7472, 3.3181)
  line L21 (1.7472, 3.3181) -> (1.0215, 2.2818)
  line L22 (2.0524, 2.8823) -> (1.6138, 2.2559)
  line L23 (-4.1637, 3.9656) -> (-1.7472, 3.3181)
  line L24 (-4.5269, 3.5453) -> (-2.0524, 2.8823)
  line L25 (-2.0524, 2.8823) -> (-1.6138, 2.2559)
  line L26 (-2.7606, 0.2696) -> (-2.1872, 1.2628)
  line L27 (-1.6138, 2.2559) -> (-2.1872, 1.2628)
  line L28 (-1.7472, 3.3181) -> (-1.0215, 2.2818)
  line L29 (-5.3338, 2.1478) -> (-3.5223, 0.3363)
  line L30 (-5.5162, 1.623) -> (-3.7472, -0.146)
  line L31 (-3.7472, -0.146) -> (-2.4868, -0.2562)
  line L32 (-3.5223, 0.3363) -> (-2.7606, 0.2696)
  dimension "d72" = 1.5
  dimension "d73" = 1.15
  dimension "d74" = 5
  dimension "d75" = 15
  dimension "d79" = 7.5
  dimension "d80" = 2
  dimension "d81" = 140
  dimension "d82" = 0.5
  dimension "d84" = 360
  constraint coincident A0.centre A1.centre
  constraint concentric A1 A2
  constraint coincident A2 L0.start
  constraint coincident A2 L1.end
  constraint vertical L1
  constraint coincident A4 L2.end
  constraint concentric A4 A5
  constraint coincident L0.end A5
  constraint coincident L1 L3.end
  constraint perpendicular L1 L3
  constraint symmetric L0.start L1 L6.start
  constraint symmetric L1 L0.end L5.start
  constraint symmetric L1 L2.end L4.start
  constraint symmetric L1 L3.end L4.end
  constraint coincident A2 L12.start
  constraint coincident A2 L7.start
  measures "d72" diameter of A1
  measures "d73" distance of A2 A3
  measures "d74" diameter of A4
  measures "d75" angle of L0 L1
  measures "d79" diameter of A5
  measures "d80" distance of L1 L0.end
  measures "d81" angle of L0 L2
extrude "Extruir16" cut sketch "Boceto15" against normal blind 1.9 contours A1 | A2 A4 L5 L6 L13 L18 | A2 L14 L15 L16 L17 L19 L22 | A2 L7 L8 L9 L10 L11 L12 | A2 A4 L20 L21 L23 L28 | A2 A4 L0 L2 L30 L31 | A2 L24 L25 L26 L27 L29 L32 bodies 4
sketch "Boceto16" plane through (0, 0, 3) normal (0, 0, -1) x (1, 0, 0)
  circle A0 centre (0, 0) radius 6.2
  circle A1 centre (0, 0) radius 6.9
  line L0 (-1.25, 6.2) -> (1.25, 6.2)
  line L1 (-1.25, 6.2) -> (-1.25, 6.0727)
  line L2 (1.25, 6.2) -> (1.25, 6.0727)
  line L3 (-4.1825, 4.7444) -> (-4.1189, 4.6341)
  line L4 (-4.1825, 4.7444) -> (-2.0175, 5.9944)
  line L5 (-2.0175, 5.9944) -> (-1.9538, 5.8841)
  line L6 (-5.9944, 2.0175) -> (-5.8841, 1.9538)
  line L7 (-5.9944, 2.0175) -> (-4.7444, 4.1825)
  line L8 (-4.7444, 4.1825) -> (-4.6341, 4.1189)
  line L9 (-6.2, -1.25) -> (-6.0727, -1.25)
  line L10 (-6.2, -1.25) -> (-6.2, 1.25)
  line L11 (-6.2, 1.25) -> (-6.0727, 1.25)
  line L12 (-4.7444, -4.1825) -> (-4.6341, -4.1189)
  line L13 (-4.7444, -4.1825) -> (-5.9944, -2.0175)
  line L14 (-5.9944, -2.0175) -> (-5.8841, -1.9538)
  line L15 (-2.0175, -5.9944) -> (-1.9538, -5.8841)
  line L16 (-2.0175, -5.9944) -> (-4.1825, -4.7444)
  line L17 (-4.1825, -4.7444) -> (-4.1189, -4.6341)
  line L18 (1.25, -6.2) -> (1.25, -6.0727)
  line L19 (1.25, -6.2) -> (-1.25, -6.2)
  line L20 (-1.25, -6.2) -> (-1.25, -6.0727)
  line L21 (4.1825, -4.7444) -> (4.1189, -4.6341)
  line L22 (4.1825, -4.7444) -> (2.0175, -5.9944)
  line L23 (2.0175, -5.9944) -> (1.9538, -5.8841)
  line L24 (5.9944, -2.0175) -> (5.8841, -1.9538)
  line L25 (5.9944, -2.0175) -> (4.7444, -4.1825)
  line L26 (4.7444, -4.1825) -> (4.6341, -4.1189)
  line L27 (6.2, 1.25) -> (6.0727, 1.25)
  line L28 (6.2, 1.25) -> (6.2, -1.25)
  line L29 (6.2, -1.25) -> (6.0727, -1.25)
  line L30 (4.7444, 4.1825) -> (4.6341, 4.1189)
  line L31 (4.7444, 4.1825) -> (5.9944, 2.0175)
  line L32 (5.9944, 2.0175) -> (5.8841, 1.9538)
  line L33 (2.0175, 5.9944) -> (1.9538, 5.8841)
  line L34 (2.0175, 5.9944) -> (4.1825, 4.7444)
  line L35 (4.1825, 4.7444) -> (4.1189, 4.6341)
  dimension "d87" = 2.5
  dimension "d88" = 1.25
  dimension "d90" = 360
  constraint horizontal L0
  constraint tangent A0 L0
  constraint coincident A0 L1.end
  constraint perpendicular L0 L1
  constraint coincident A0 L2.end
  constraint perpendicular L0 L2
  measures "d87" distance of L0.start L0.end
  measures "d88" horizontal distance of A0.centre L0.start
extrude "Extruir17" cut sketch "Boceto16" against normal blind 3 contours A0 L28 L29 | A0 L27 L28 | A0 L31 L32 | A0 L24 L25 | A0 L30 L31 | A0 L25 L26 | A0 L34 L35 | A0 L21 L22 | A0 L33 L34 | A0 L22 L23 | A0 L0 L2 | A0 L18 L19 | A0 L0 L1 | A0 L19 L20 | A0 L4 L5 | A0 L15 L16 | A0 L3 L4 | A0 L16 L17 | A0 L7 L8 | A0 L12 L13 | A0 L6 L7 | A0 L13 L14 | A0 L10 L11 | A0 L9 L10 bodies 4
fillet "Empalme1" radius 0.5 18 edges at (-4.1637, -3.9656, 7.2269) (-5.5162, -1.623, 7.2269) (4.1637, -3.9656, 7.2269) (5.5162, -1.623, 7.2269) (1.0215, -2.2818, 8.3379) (-1.0215, -2.2818, 8.3379) (-1.3525, 5.5887, 7.2269) (1.3525, 5.5887, 7.2269) (-5.3338, -2.1478, 7.2269) (-4.5269, -3.5453, 7.2269) (4.5269, -3.5453, 7.2269) (5.3338, -2.1478, 7.2269) (0.8069, 5.6931, 7.2269) (-0.8069, 5.6931, 7.2269) (-1.4653, 2.0255, 8.3379) (-2.4868, 0.2562, 8.3379) (1.4653, 2.0255, 8.3379) (2.4868, 0.2562, 8.3379) on bodies 4
chamfer "Chaflán1" distance 0.2 angle 45 2 edges at (-0.6992, -0.2712, 13.75) (-0.6992, 0.2712, -0.5) tangent chain off on bodies 3
copy_body "Cuerpo - > Comp.1" bodies 1 removing the originals makes body 17 in component "Component"
copy_body "Cuerpo - > Comp.2" bodies 2 removing the originals makes body 18 in component "Component'"
copy_body "Cuerpo - > Comp.3" bodies 3 removing the originals makes body 19 in component "Component''"
copy_body "Cuerpo - > Comp.4" bodies 4 removing the originals makes body 20 in component "Component'''"
copy_body "Cuerpo - > Comp.5" bodies 5 removing the originals makes body 21 in component "Component''''"
copy_body "Cuerpo - > Comp.6" bodies 6 removing the originals makes body 22 in component "Component'''''"
copy_body "Cuerpo - > Comp.7" bodies 7 removing the originals makes body 23 in component "Component''''''"
copy_body "Cuerpo - > Comp.8" bodies 8 removing the originals makes body 24 in component "Component'''''''"
copy_body "Cuerpo - > Comp.9" bodies 9 removing the originals makes body 25 in component "Component''''''''"
copy_body "Cuerpo - > Comp.10" bodies 10 removing the originals makes body 26 in component "Component'''''''''"
copy_body "Cuerpo - > Comp.11" bodies 11 removing the originals makes body 27 in component "Component''''''''''"
copy_body "Cuerpo - > Comp.12" bodies 12 removing the originals makes body 28 in component "Component'''''''''''"
copy_body "Cuerpo - > Comp.13" bodies 13 removing the originals makes body 29 in component "Component''''''''''''"
copy_body "Cuerpo - > Comp.14" bodies 14 removing the originals makes body 30 in component "Component'''''''''''''"
copy_body "Cuerpo - > Comp.15" bodies 15 removing the originals makes body 31 in component "Component''''''''''''''"
copy_body "Cuerpo - > Comp.16" bodies 16 removing the originals makes body 32 in component "Component'''''''''''''''"
component "Component" placed x (1, 0, 0) y (0, 1, 0) z (0, 0, 1) at (0, 0, 0)
component "Component'" placed x (1, 0, 0) y (0, 1, 0) z (0, 0, 1) at (0, 0, 0)
component "Component''" placed x (1, 0, 0) y (0, 1, 0) z (0, 0, 1) at (0, 0, 0)
component "Component'''" placed x (1, 0, 0) y (0, 1, 0) z (0, 0, 1) at (0, 0, 0)
component "Component''''" placed x (-1, 0, 0) y (0, -1, 0) z (0, 0, 1) at (0, -11.7, 0)
component "Component'''''" placed x (-1, 0, 0) y (0, -1, 0) z (0, 0, 1) at (5.85, -10.1325, 0)
component "Component''''''" placed x (-1, 0, 0) y (0, -1, 0) z (0, 0, 1) at (10.1325, -5.85, 0)
component "Component'''''''" placed x (-1, 0, 0) y (0, -1, 0) z (0, 0, 1) at (11.7, 0, 0)
component "Component''''''''" placed x (-1, 0, 0) y (0, -1, 0) z (0, 0, 1) at (10.1325, 5.85, 0)
component "Component'''''''''" placed x (-1, 0, 0) y (0, -1, 0) z (0, 0, 1) at (5.85, 10.1325, 0)
component "Component''''''''''" placed x (-1, 0, 0) y (0, -1, 0) z (0, 0, 1) at (0, 11.7, 0)
component "Component'''''''''''" placed x (-1, 0, 0) y (0, -1, 0) z (0, 0, 1) at (-5.85, 10.1325, 0)
component "Component''''''''''''" placed x (-1, 0, 0) y (0, -1, 0) z (0, 0, 1) at (-10.1325, 5.85, 0)
component "Component'''''''''''''" placed x (-1, 0, 0) y (0, -1, 0) z (0, 0, 1) at (-11.7, 0, 0)
component "Component''''''''''''''" placed x (-1, 0, 0) y (0, -1, 0) z (0, 0, 1) at (-10.1325, -5.85, 0)
component "Component'''''''''''''''" placed x (-1, 0, 0) y (0, -1, 0) z (0, 0, 1) at (-5.85, -10.1325, 0)
equation "d22 = -14.25 mm + 0.5 mm"
equation "d37 = d36 / 2"
equation "d58 = d56 / 2"
equation "d88 = d87 / 2"
